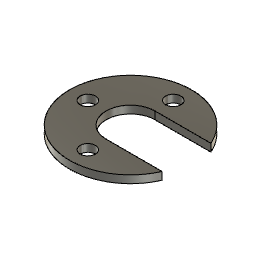
Model 6 (Autodesk Fusion 360 design; units mm, degrees)
Autodesk Fusion 360 part; units mm, degrees
sketch "Sketch1" plane through (0, 0, 0) normal (0, 0, 1) x (1, 0, 0)
  line L0 (36.6606, 16) -> (0, 16)
  line L1 (0, -16) -> (36.6606, -16)
  arc A0 (0, 16) -> (0, -16) centre (0, 0) ccw
  arc A1 (36.6606, 16) -> (36.6606, -16) centre (0, 0) ccw
  dimension "d1" = 32
  dimension "d2" = 80
  constraint coincident A0.centre A1.centre
  constraint tangent L0 A0
  measures "d1" diameter of A0
  measures "d2" diameter of A1
extrude "Extrude1" add sketch "Sketch1" along normal blind 5
sketch "Sketch2" plane through (0, 0, 5) normal (0, 0, 1) x (-1, 0, 0)
  line L0 (0, -16) -> (-36.6606, -16)
  arc A0 (-36.6606, -16) -> (-36.6606, 16) centre (0, 0) ccw
  line L1 (-36.6606, 16) -> (0, 16)
  arc A1 (0, -16) -> (0, 16) centre (0, 0) ccw
  line L2 (0, 0) -> (0, -28) construction
  circle A2 centre (0, -28) radius 5
  circle A3 centre (28, 0) radius 5
  circle A4 centre (0, 28) radius 5
  dimension "d5" = 28
  dimension "d6" = 10
  dimension "d8" = 180
  constraint coincident A0.centre A1.centre
  constraint vertical L2
  constraint coincident L2.end A2.centre
  measures "d5" distance of A0.centre L2.end
  measures "d6" diameter of A2
extrude "Extrude2" cut sketch "Sketch2" against normal blind 5 contours A2 | A3 | A4
